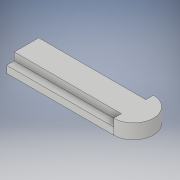
# Autodesk Inventor part: tenshoner slider
Saved by Autodesk Inventor 2019 (Build 230136000, 136)
## iProperties
Created: 2019-12-07
Part Number: tenshoner slider
Material: Generic
Document SubType Name: Modeling
Designer: User
Density: 1 g/cm^3
Appearance: Default
Author: User
Autodesk Inventor part; units mm, degrees
ref_plane "YZ Plane" through (0, 0, 0) normal (1, 0, 0) x (0, 1, 0)
ref_plane "XZ Plane" through (0, 0, 0) normal (0, 1, 0) x (-1, 0, 0)
ref_plane "XY Plane" through (0, 0, 0) normal (0, 0, 1) x (1, 0, 0)
sketch "Sketch1" plane through (0, 0, 0) normal (1, 0, 0) x (0, 1, 0)
  line L0 (0, 0) -> (2.921, 0)
  line L1 (2.921, 0) -> (2.921, -16.51)
  line L2 (2.921, -16.51) -> (0, -16.51)
  line L3 (0, -16.51) -> (0, 0)
  line L4 (2.921, -3.175) -> (6.096, -3.175)
  line L5 (6.096, -3.175) -> (6.096, -13.335)
  line L6 (6.096, -13.335) -> (2.921, -13.335)
  line L7 (2.921, -13.335) -> (2.921, -3.175)
  dimension "d0" = 16.51
  dimension "d1" = 10.16
  dimension "d2" = 3.175
  dimension "d3" = 2.921
  dimension "d4" = 3.175
  constraints: 16 end point, 4 parallel, 2 horizontal, 2 perpendicular, 1 point on line
  measures "d0" distance of L2.end L0.start
  measures "d1" distance between parallel lines of L6 L4
  measures "d2" distance between parallel lines of L2 L6
  measures "d3" distance between parallel lines of L3 L1
  measures "d4" distance between parallel lines of L1 L5
extrude "Extrusion1" add sketch "Sketch1" along normal blind 44.45
sketch "Sketch2" plane through (0, 0, -16.51) normal (0, -1, 0) x (1, 0, 0)
  line L0 (44.45, 16.51) -> (44.45, 0) projected
  arc A0 (44.45, 0) -> (44.45, 16.51) centre (44.45, 8.255) ccw
  point P0 (0, 16.51)
  constraints: 2 point on circle, 1 centre point
extrude "Extrusion2" add sketch "Sketch2" against normal up to surface (6.096 mm away)
equation "\"d2\" = -0.5 * d1 + 0.5 * d0"
body "Solid1"
